Autodesk Fusion 360 part; units mm, degrees
(part 2 of 5)
sketch "Sketch7" plane through (0, 0, -0.05) normal (0, 0, -1) x (1, 0, 0)
  arc A0 (124.5324, 39.9718) -> (129.3118, 35.1924) centre (129.53, 40.19) ccw
  line L0 (129.3118, 35.1924) -> (129.53, 35.19)
  line L1 (129.53, 35.19) -> (210.09, 35.19)
  line L2 (210.09, 35.19) -> (210.3082, 35.1924)
  arc A1 (210.3082, 35.1924) -> (215.0876, 39.9718) centre (210.09, 40.19) ccw
  line L3 (215.0876, 39.9718) -> (215.09, 40.19)
  line L4 (215.09, 40.19) -> (215.09, 102.8)
  line L5 (215.09, 102.8) -> (215.0877, 103.0182)
  arc A2 (215.0877, 103.0182) -> (210.3082, 107.7977) centre (210.09, 102.8) ccw
  line L6 (210.3082, 107.7977) -> (210.09, 107.8)
  line L7 (210.09, 107.8) -> (129.53, 107.8)
  line L8 (129.53, 107.8) -> (129.3118, 107.7977)
  arc A3 (129.3118, 107.7977) -> (124.5323, 103.0182) centre (129.53, 102.8) ccw
  line L9 (124.5323, 103.0182) -> (124.53, 102.8)
  line L10 (124.53, 102.8) -> (124.53, 40.19)
  line L11 (124.53, 40.19) -> (124.5324, 39.9718)
  circle A4 centre (172, 103.08) radius 1.077
  circle A5 centre (184.5, 103.08) radius 1.077
  circle A6 centre (129.53, 102.8) radius 1.3
  circle A7 centre (210.09, 102.8) radius 1.3
  arc A8 (172.975, 97.003) -> (173.077, 97.105) centre (172.975, 97.105) ccw
  line L12 (172.975, 97.003) -> (171.025, 97.003)
  arc A9 (170.923, 97.105) -> (171.025, 97.003) centre (171.025, 97.105) ccw
  line L13 (170.923, 97.105) -> (170.923, 99.055)
  arc A10 (171.025, 99.157) -> (170.923, 99.055) centre (171.025, 99.055) ccw
  line L14 (171.025, 99.157) -> (172.975, 99.157)
  arc A11 (173.077, 99.055) -> (172.975, 99.157) centre (172.975, 99.055) ccw
  line L15 (173.077, 99.055) -> (173.077, 97.105)
  circle A12 centre (184.5, 98.08) radius 1.077
  line L16 (212.43, 78.91) -> (212.43, 77.21)
  line L17 (212.43, 77.21) -> (210.73, 77.21)
  line L18 (210.73, 77.21) -> (210.73, 78.91)
  line L19 (210.73, 78.91) -> (212.43, 78.91)
  circle A13 centre (211.58, 75.52) radius 0.85
  circle A14 centre (211.58, 72.98) radius 0.85
  circle A15 centre (211.58, 70.44) radius 0.85
  circle A16 centre (211.58, 67.9) radius 0.85
  circle A17 centre (211.58, 65.36) radius 0.85
  circle A18 centre (211.58, 62.82) radius 0.85
  circle A19 centre (211.58, 60.28) radius 0.85
  arc A20 (164.6391, 57.504) -> (164.7411, 57.606) centre (164.6391, 57.606) ccw
  line L20 (164.6391, 57.504) -> (162.6391, 57.504)
  arc A21 (162.5371, 57.606) -> (162.6391, 57.504) centre (162.6391, 57.606) ccw
  line L21 (162.5371, 57.606) -> (162.5371, 59.114)
  arc A22 (162.6391, 59.216) -> (162.5371, 59.114) centre (162.6391, 59.114) ccw
  line L22 (162.6391, 59.216) -> (164.6391, 59.216)
  arc A23 (164.7411, 59.114) -> (164.6391, 59.216) centre (164.6391, 59.114) ccw
  line L23 (164.7411, 59.114) -> (164.7411, 57.606)
  arc A24 (182.0197, 57.504) -> (182.1217, 57.606) centre (182.0197, 57.606) ccw
  line L24 (182.0197, 57.504) -> (180.0197, 57.504)
  arc A25 (179.9177, 57.606) -> (180.0197, 57.504) centre (180.0197, 57.606) ccw
  line L25 (179.9177, 57.606) -> (179.9177, 59.114)
  arc A26 (180.0197, 59.216) -> (179.9177, 59.114) centre (180.0197, 59.114) ccw
  line L26 (180.0197, 59.216) -> (182.0197, 59.216)
  arc A27 (182.1217, 59.114) -> (182.0197, 59.216) centre (182.0197, 59.114) ccw
  line L27 (182.1217, 59.114) -> (182.1217, 57.606)
  circle A28 centre (211.58, 57.74) radius 0.85
  arc A29 (164.6322, 54.964) -> (164.7342, 55.066) centre (164.6322, 55.066) ccw
  line L28 (164.6322, 54.964) -> (162.6322, 54.964)
  arc A30 (162.5302, 55.066) -> (162.6322, 54.964) centre (162.6322, 55.066) ccw
  line L29 (162.5302, 55.066) -> (162.5302, 56.574)
  arc A31 (162.6322, 56.676) -> (162.5302, 56.574) centre (162.6322, 56.574) ccw
  line L30 (162.6322, 56.676) -> (164.6322, 56.676)
  arc A32 (164.7342, 56.574) -> (164.6322, 56.676) centre (164.6322, 56.574) ccw
  line L31 (164.7342, 56.574) -> (164.7342, 55.066)
  arc A33 (182.0197, 54.964) -> (182.1217, 55.066) centre (182.0197, 55.066) ccw
  line L32 (182.0197, 54.964) -> (180.0197, 54.964)
  arc A34 (179.9177, 55.066) -> (180.0197, 54.964) centre (180.0197, 55.066) ccw
  line L33 (179.9177, 55.066) -> (179.9177, 56.574)
  arc A35 (180.0197, 56.676) -> (179.9177, 56.574) centre (180.0197, 56.574) ccw
  line L34 (180.0197, 56.676) -> (182.0197, 56.676)
  arc A36 (182.1217, 56.574) -> (182.0197, 56.676) centre (182.0197, 56.574) ccw
  line L35 (182.1217, 56.574) -> (182.1217, 55.066)
  circle A37 centre (211.58, 55.2) radius 0.85
  arc A38 (199.24, 52.73) -> (199.49, 52.98) centre (199.24, 52.98) ccw
  line L36 (199.24, 52.73) -> (198.59, 52.73)
  arc A39 (198.34, 52.98) -> (198.59, 52.73) centre (198.59, 52.98) ccw
  line L37 (198.34, 52.98) -> (198.34, 54.28)
  arc A40 (198.59, 54.53) -> (198.34, 54.28) centre (198.59, 54.28) ccw
  line L38 (198.59, 54.53) -> (199.24, 54.53)
  arc A41 (199.49, 54.28) -> (199.24, 54.53) centre (199.24, 54.28) ccw
  line L39 (199.49, 54.28) -> (199.49, 52.98)
  arc A42 (202.19, 52.73) -> (202.44, 52.98) centre (202.19, 52.98) ccw
  line L40 (202.19, 52.73) -> (201.54, 52.73)
  arc A43 (201.29, 52.98) -> (201.54, 52.73) centre (201.54, 52.98) ccw
  line L41 (201.29, 52.98) -> (201.29, 54.28)
  arc A44 (201.54, 54.53) -> (201.29, 54.28) centre (201.54, 54.28) ccw
  line L42 (201.54, 54.53) -> (202.19, 54.53)
  arc A45 (202.44, 54.28) -> (202.19, 54.53) centre (202.19, 54.28) ccw
  line L43 (202.44, 54.28) -> (202.44, 52.98)
  arc A46 (164.6322, 52.424) -> (164.7342, 52.526) centre (164.6322, 52.526) ccw
  line L44 (164.6322, 52.424) -> (162.6322, 52.424)
  arc A47 (162.5302, 52.526) -> (162.6322, 52.424) centre (162.6322, 52.526) ccw
  line L45 (162.5302, 52.526) -> (162.5302, 54.034)
  arc A48 (162.6322, 54.136) -> (162.5302, 54.034) centre (162.6322, 54.034) ccw
  line L46 (162.6322, 54.136) -> (164.6322, 54.136)
  arc A49 (164.7342, 54.034) -> (164.6322, 54.136) centre (164.6322, 54.034) ccw
  line L47 (164.7342, 54.034) -> (164.7342, 52.526)
  arc A50 (182.0197, 52.424) -> (182.1217, 52.526) centre (182.0197, 52.526) ccw
  line L48 (182.0197, 52.424) -> (180.0197, 52.424)
  arc A51 (179.9177, 52.526) -> (180.0197, 52.424) centre (180.0197, 52.526) ccw
  line L49 (179.9177, 52.526) -> (179.9177, 54.034)
  arc A52 (180.0197, 54.136) -> (179.9177, 54.034) centre (180.0197, 54.034) ccw
  line L50 (180.0197, 54.136) -> (182.0197, 54.136)
  arc A53 (182.1217, 54.034) -> (182.0197, 54.136) centre (182.0197, 54.034) ccw
  line L51 (182.1217, 54.034) -> (182.1217, 52.526)
  circle A54 centre (211.58, 52.66) radius 0.85
  arc A55 (164.6322, 49.884) -> (164.7342, 49.986) centre (164.6322, 49.986) ccw
  line L52 (164.6322, 49.884) -> (162.6322, 49.884)
  arc A56 (162.5302, 49.986) -> (162.6322, 49.884) centre (162.6322, 49.986) ccw
  line L53 (162.5302, 49.986) -> (162.5302, 51.494)
  arc A57 (162.6322, 51.596) -> (162.5302, 51.494) centre (162.6322, 51.494) ccw
  line L54 (162.6322, 51.596) -> (164.6322, 51.596)
  arc A58 (164.7342, 51.494) -> (164.6322, 51.596) centre (164.6322, 51.494) ccw
  line L55 (164.7342, 51.494) -> (164.7342, 49.986)
  arc A59 (182.0197, 49.884) -> (182.1217, 49.986) centre (182.0197, 49.986) ccw
  line L56 (182.0197, 49.884) -> (180.0197, 49.884)
  arc A60 (179.9177, 49.986) -> (180.0197, 49.884) centre (180.0197, 49.986) ccw
  line L57 (179.9177, 49.986) -> (179.9177, 51.494)
  arc A61 (180.0197, 51.596) -> (179.9177, 51.494) centre (180.0197, 51.494) ccw
  line L58 (180.0197, 51.596) -> (182.0197, 51.596)
  arc A62 (182.1217, 51.494) -> (182.0197, 51.596) centre (182.0197, 51.494) ccw
  line L59 (182.1217, 51.494) -> (182.1217, 49.986)
  line L60 (140.26, 51.04) -> (140.26, 49.44)
  line L61 (140.26, 49.44) -> (139.56, 49.44)
  line L62 (139.56, 49.44) -> (139.56, 51.04)
  line L63 (139.56, 51.04) -> (140.26, 51.04)
  line L64 (141.36, 51.04) -> (141.36, 49.44)
  line L65 (141.36, 49.44) -> (140.66, 49.44)
  line L66 (140.66, 49.44) -> (140.66, 51.04)
  line L67 (140.66, 51.04) -> (141.36, 51.04)
  line L68 (142.46, 51.04) -> (142.46, 49.44)
  line L69 (142.46, 49.44) -> (141.76, 49.44)
  line L70 (141.76, 49.44) -> (141.76, 51.04)
  line L71 (141.76, 51.04) -> (142.46, 51.04)
  line L72 (143.56, 51.04) -> (143.56, 49.44)
  line L73 (143.56, 49.44) -> (142.86, 49.44)
  line L74 (142.86, 49.44) -> (142.86, 51.04)
  line L75 (142.86, 51.04) -> (143.56, 51.04)
  line L76 (144.66, 51.04) -> (144.66, 49.44)
  line L77 (144.66, 49.44) -> (143.96, 49.44)
  line L78 (143.96, 49.44) -> (143.96, 51.04)
  line L79 (143.96, 51.04) -> (144.66, 51.04)
  line L80 (145.76, 51.04) -> (145.76, 49.44)
  line L81 (145.76, 49.44) -> (145.06, 49.44)
  line L82 (145.06, 49.44) -> (145.06, 51.04)
  line L83 (145.06, 51.04) -> (145.76, 51.04)
  line L84 (146.86, 51.04) -> (146.86, 49.44)
  line L85 (146.86, 49.44) -> (146.16, 49.44)
  line L86 (146.16, 49.44) -> (146.16, 51.04)
  line L87 (146.16, 51.04) -> (146.86, 51.04)
  line L88 (147.96, 51.04) -> (147.96, 49.44)
  line L89 (147.96, 49.44) -> (147.26, 49.44)
  line L90 (147.26, 49.44) -> (147.26, 51.04)
  line L91 (147.26, 51.04) -> (147.96, 51.04)
  line L92 (149.06, 51.04) -> (149.06, 49.44)
  line L93 (149.06, 49.44) -> (148.36, 49.44)
  line L94 (148.36, 49.44) -> (148.36, 51.04)
  line L95 (148.36, 51.04) -> (149.06, 51.04)
  circle A63 centre (211.58, 50.12) radius 0.85
  line L96 (139.26, 49.99) -> (139.26, 48.49)
  line L97 (139.26, 48.49) -> (138.06, 48.49)
  line L98 (138.06, 48.49) -> (138.06, 49.99)
  line L99 (138.06, 49.99) -> (139.26, 49.99)
  line L100 (154.11, 49.99) -> (154.11, 48.49)
  line L101 (154.11, 48.49) -> (152.51, 48.49)
  line L102 (152.51, 48.49) -> (152.51, 49.99)
  line L103 (152.51, 49.99) -> (154.11, 49.99)
  arc A64 (164.6322, 47.344) -> (164.7342, 47.446) centre (164.6322, 47.446) ccw
  line L104 (164.6322, 47.344) -> (162.6322, 47.344)
  arc A65 (162.5302, 47.446) -> (162.6322, 47.344) centre (162.6322, 47.446) ccw
  line L105 (162.5302, 47.446) -> (162.5302, 48.954)
  arc A66 (162.6322, 49.056) -> (162.5302, 48.954) centre (162.6322, 48.954) ccw
  line L106 (162.6322, 49.056) -> (164.6322, 49.056)
  arc A67 (164.7342, 48.954) -> (164.6322, 49.056) centre (164.6322, 48.954) ccw
  line L107 (164.7342, 48.954) -> (164.7342, 47.446)
  arc A68 (182.0197, 47.344) -> (182.1217, 47.446) centre (182.0197, 47.446) ccw
  line L108 (182.0197, 47.344) -> (180.0197, 47.344)
  arc A69 (179.9177, 47.446) -> (180.0197, 47.344) centre (180.0197, 47.446) ccw
  line L109 (179.9177, 47.446) -> (179.9177, 48.954)
  arc A70 (180.0197, 49.056) -> (179.9177, 48.954) centre (180.0197, 48.954) ccw
  line L110 (180.0197, 49.056) -> (182.0197, 49.056)
  arc A71 (182.1217, 48.954) -> (182.0197, 49.056) centre (182.0197, 48.954) ccw
  line L111 (182.1217, 48.954) -> (182.1217, 47.446)
  circle A72 centre (211.58, 47.58) radius 0.85
  circle A73 centre (196.89, 46.1501) radius 0.6604
  circle A74 centre (199.43, 46.1501) radius 0.6604
  circle A75 centre (201.97, 46.1501) radius 0.6604
  arc A76 (164.6322, 44.804) -> (164.7342, 44.906) centre (164.6322, 44.906) ccw
  line L112 (164.6322, 44.804) -> (162.6322, 44.804)
  arc A77 (162.5302, 44.906) -> (162.6322, 44.804) centre (162.6322, 44.906) ccw
  line L113 (162.5302, 44.906) -> (162.5302, 46.414)
  arc A78 (162.6322, 46.516) -> (162.5302, 46.414) centre (162.6322, 46.414) ccw
  line L114 (162.6322, 46.516) -> (164.6322, 46.516)
  arc A79 (164.7342, 46.414) -> (164.6322, 46.516) centre (164.6322, 46.414) ccw
  line L115 (164.7342, 46.414) -> (164.7342, 44.906)
  arc A80 (182.0197, 44.804) -> (182.1217, 44.906) centre (182.0197, 44.906) ccw
  line L116 (182.0197, 44.804) -> (180.0197, 44.804)
  arc A81 (179.9177, 44.906) -> (180.0197, 44.804) centre (180.0197, 44.906) ccw
  line L117 (179.9177, 44.906) -> (179.9177, 46.414)
  arc A82 (180.0197, 46.516) -> (179.9177, 46.414) centre (180.0197, 46.414) ccw
  line L118 (180.0197, 46.516) -> (182.0197, 46.516)
  arc A83 (182.1217, 46.414) -> (182.0197, 46.516) centre (182.0197, 46.414) ccw
  line L119 (182.1217, 46.414) -> (182.1217, 44.906)
  circle A84 centre (211.58, 45.04) radius 0.85
  arc A85 (164.6322, 42.264) -> (164.7342, 42.366) centre (164.6322, 42.366) ccw
  line L120 (164.6322, 42.264) -> (162.6322, 42.264)
  arc A86 (162.5302, 42.366) -> (162.6322, 42.264) centre (162.6322, 42.366) ccw
  line L121 (162.5302, 42.366) -> (162.5302, 43.874)
  arc A87 (162.6322, 43.976) -> (162.5302, 43.874) centre (162.6322, 43.874) ccw
  line L122 (162.6322, 43.976) -> (164.6322, 43.976)
  arc A88 (164.7342, 43.874) -> (164.6322, 43.976) centre (164.6322, 43.874) ccw
  line L123 (164.7342, 43.874) -> (164.7342, 42.366)
  arc A89 (182.0197, 42.264) -> (182.1217, 42.366) centre (182.0197, 42.366) ccw
  line L124 (182.0197, 42.264) -> (180.0197, 42.264)
  arc A90 (179.9177, 42.366) -> (180.0197, 42.264) centre (180.0197, 42.366) ccw
  line L125 (179.9177, 42.366) -> (179.9177, 43.874)
  arc A91 (180.0197, 43.976) -> (179.9177, 43.874) centre (180.0197, 43.874) ccw
  line L126 (180.0197, 43.976) -> (182.0197, 43.976)
  arc A92 (182.1217, 43.874) -> (182.0197, 43.976) centre (182.0197, 43.874) ccw
  line L127 (182.1217, 43.874) -> (182.1217, 42.366)
  circle A93 centre (129.53, 40.19) radius 1.3
  circle A94 centre (210.09, 40.19) radius 1.3
  arc A95 (164.6322, 39.724) -> (164.7342, 39.826) centre (164.6322, 39.826) ccw
  line L128 (164.6322, 39.724) -> (162.6322, 39.724)
  arc A96 (162.5302, 39.826) -> (162.6322, 39.724) centre (162.6322, 39.826) ccw
  line L129 (162.5302, 39.826) -> (162.5302, 41.334)
  arc A97 (162.6322, 41.436) -> (162.5302, 41.334) centre (162.6322, 41.334) ccw
  line L130 (162.6322, 41.436) -> (164.6322, 41.436)
  arc A98 (164.7342, 41.334) -> (164.6322, 41.436) centre (164.6322, 41.334) ccw
  line L131 (164.7342, 41.334) -> (164.7342, 39.826)
  arc A99 (182.0197, 39.724) -> (182.1217, 39.826) centre (182.0197, 39.826) ccw
  line L132 (182.0197, 39.724) -> (180.0197, 39.724)
  arc A100 (179.9177, 39.826) -> (180.0197, 39.724) centre (180.0197, 39.826) ccw
  line L133 (179.9177, 39.826) -> (179.9177, 41.334)
  arc A101 (180.0197, 41.436) -> (179.9177, 41.334) centre (180.0197, 41.334) ccw
  line L134 (180.0197, 41.436) -> (182.0197, 41.436)
  arc A102 (182.1217, 41.334) -> (182.0197, 41.436) centre (182.0197, 41.334) ccw
  line L135 (182.1217, 41.334) -> (182.1217, 39.826)
  line L136 (139.26, 40.74) -> (139.26, 38.54)
  line L137 (139.26, 38.54) -> (138.06, 38.54)
  line L138 (138.06, 38.54) -> (138.06, 40.74)
  line L139 (138.06, 40.74) -> (139.26, 40.74)
  line L140 (154.86, 40.74) -> (154.86, 38.54)
  line L141 (154.86, 38.54) -> (153.66, 38.54)
  line L142 (153.66, 38.54) -> (153.66, 40.74)
  line L143 (153.66, 40.74) -> (154.86, 40.74)
  arc A103 (164.6322, 37.184) -> (164.7342, 37.286) centre (164.6322, 37.286) ccw
  line L144 (164.6322, 37.184) -> (162.6322, 37.184)
  arc A104 (162.5302, 37.286) -> (162.6322, 37.184) centre (162.6322, 37.286) ccw
  line L145 (162.5302, 37.286) -> (162.5302, 38.794)
  arc A105 (162.6322, 38.896) -> (162.5302, 38.794) centre (162.6322, 38.794) ccw
  line L146 (162.6322, 38.896) -> (164.6322, 38.896)
  arc A106 (164.7342, 38.794) -> (164.6322, 38.896) centre (164.6322, 38.794) ccw
  line L147 (164.7342, 38.794) -> (164.7342, 37.286)
  arc A107 (182.0197, 37.184) -> (182.1217, 37.286) centre (182.0197, 37.286) ccw
  line L148 (182.0197, 37.184) -> (180.0197, 37.184)
  arc A108 (179.9177, 37.286) -> (180.0197, 37.184) centre (180.0197, 37.286) ccw
  line L149 (179.9177, 37.286) -> (179.9177, 38.794)
  arc A109 (180.0197, 38.896) -> (179.9177, 38.794) centre (180.0197, 38.794) ccw
  line L150 (180.0197, 38.896) -> (182.0197, 38.896)
  arc A110 (182.1217, 38.794) -> (182.0197, 38.896) centre (182.0197, 38.794) ccw
  line L151 (182.1217, 38.794) -> (182.1217, 37.286)
  circle A111 centre (129.53, 102.8) radius 6.8089
  circle A112 centre (129.53, 40.19) radius 7.6352
  spline S0 degree 5 poles (207.5436, 38.5257) (207.5062, 38.7717) (207.4443, 39.2717) (207.3918, 40.0335) (207.4207, 41.0207) (207.6971, 42.0707) (208.2833, 42.8142) (209.2088, 43.1592) (210.4206, 43.0662) (211.7646, 42.5596) (213.0388, 41.708) (214.0308, 40.6116) (214.5637, 39.3872) (214.5339, 38.1559) (213.9669, 37.0286) (212.9954, 36.1) (211.807, 35.4469) (210.6011, 35.1248) (209.5472, 35.1641) (208.7311, 35.5656) (208.1502, 36.299) (207.8391, 37.1051) (207.6691, 37.7955) (207.5811, 38.2796) (207.5436, 38.5257) knots 0 0 0 0 0 0 0.05 0.1 0.15 0.2 0.25 0.3 0.35 0.4 0.45 0.5 0.55 0.6 0.65 0.7 0.75 0.8 0.85 0.9 0.95 1 1 1 1 1 1
  point P0 (209, 43)
  point P1 (214.4745, 39.0133)
  point P2 (210.09, 35.19)
  constraint concentric A3 A111
  constraint concentric A0 A112
  constraint coincident P2 L1.end
extrude "Extrude6" add sketch "Sketch7" along normal blind 20.6 contours L2 A1 S0 | A94 picked at (207.9612, 39.4019)
sketch "Sketch8" plane through (0, 0, -0.05) normal (0, 0, -1) x (1, 0, 0)
  arc A0 (124.5324, 39.9718) -> (129.3118, 35.1924) centre (129.53, 40.19) ccw
  line L0 (129.3118, 35.1924) -> (129.53, 35.19)
  line L1 (129.53, 35.19) -> (210.09, 35.19)
  line L2 (210.09, 35.19) -> (210.3082, 35.1924)
  arc A1 (210.3082, 35.1924) -> (215.0876, 39.9718) centre (210.09, 40.19) ccw
  line L3 (215.0876, 39.9718) -> (215.09, 40.19)
  line L4 (215.09, 40.19) -> (215.09, 102.8)
  line L5 (215.09, 102.8) -> (215.0877, 103.0182)
  arc A2 (215.0877, 103.0182) -> (210.3082, 107.7977) centre (210.09, 102.8) ccw
  line L6 (210.3082, 107.7977) -> (210.09, 107.8)
  line L7 (210.09, 107.8) -> (129.53, 107.8)
  line L8 (129.53, 107.8) -> (129.3118, 107.7977)
  arc A3 (129.3118, 107.7977) -> (124.5323, 103.0182) centre (129.53, 102.8) ccw
  line L9 (124.5323, 103.0182) -> (124.53, 102.8)
  line L10 (124.53, 102.8) -> (124.53, 40.19)
  line L11 (124.53, 40.19) -> (124.5324, 39.9718)
  circle A4 centre (172, 103.08) radius 1.077
  circle A5 centre (184.5, 103.08) radius 1.077
  circle A6 centre (129.53, 102.8) radius 1.3
  circle A7 centre (210.09, 102.8) radius 1.3
  arc A8 (172.975, 97.003) -> (173.077, 97.105) centre (172.975, 97.105) ccw
  line L12 (172.975, 97.003) -> (171.025, 97.003)
  arc A9 (170.923, 97.105) -> (171.025, 97.003) centre (171.025, 97.105) ccw
  line L13 (170.923, 97.105) -> (170.923, 99.055)
  arc A10 (171.025, 99.157) -> (170.923, 99.055) centre (171.025, 99.055) ccw
  line L14 (171.025, 99.157) -> (172.975, 99.157)
  arc A11 (173.077, 99.055) -> (172.975, 99.157) centre (172.975, 99.055) ccw
  line L15 (173.077, 99.055) -> (173.077, 97.105)
  circle A12 centre (184.5, 98.08) radius 1.077
  line L16 (212.43, 78.91) -> (212.43, 77.21)
  line L17 (212.43, 77.21) -> (210.73, 77.21)
  line L18 (210.73, 77.21) -> (210.73, 78.91)
  line L19 (210.73, 78.91) -> (212.43, 78.91)
  circle A13 centre (211.58, 75.52) radius 0.85
  circle A14 centre (211.58, 72.98) radius 0.85
  circle A15 centre (211.58, 70.44) radius 0.85
  circle A16 centre (211.58, 67.9) radius 0.85
  circle A17 centre (211.58, 65.36) radius 0.85
  circle A18 centre (211.58, 62.82) radius 0.85
  circle A19 centre (211.58, 60.28) radius 0.85
  arc A20 (164.6391, 57.504) -> (164.7411, 57.606) centre (164.6391, 57.606) ccw
  line L20 (164.6391, 57.504) -> (162.6391, 57.504)
  arc A21 (162.5371, 57.606) -> (162.6391, 57.504) centre (162.6391, 57.606) ccw
  line L21 (162.5371, 57.606) -> (162.5371, 59.114)
  arc A22 (162.6391, 59.216) -> (162.5371, 59.114) centre (162.6391, 59.114) ccw
  line L22 (162.6391, 59.216) -> (164.6391, 59.216)
  arc A23 (164.7411, 59.114) -> (164.6391, 59.216) centre (164.6391, 59.114) ccw
  line L23 (164.7411, 59.114) -> (164.7411, 57.606)
  arc A24 (182.0197, 57.504) -> (182.1217, 57.606) centre (182.0197, 57.606) ccw
  line L24 (182.0197, 57.504) -> (180.0197, 57.504)
  arc A25 (179.9177, 57.606) -> (180.0197, 57.504) centre (180.0197, 57.606) ccw
  line L25 (179.9177, 57.606) -> (179.9177, 59.114)
  arc A26 (180.0197, 59.216) -> (179.9177, 59.114) centre (180.0197, 59.114) ccw
  line L26 (180.0197, 59.216) -> (182.0197, 59.216)
  arc A27 (182.1217, 59.114) -> (182.0197, 59.216) centre (182.0197, 59.114) ccw
  line L27 (182.1217, 59.114) -> (182.1217, 57.606)
  circle A28 centre (211.58, 57.74) radius 0.85
  arc A29 (164.6322, 54.964) -> (164.7342, 55.066) centre (164.6322, 55.066) ccw
  line L28 (164.6322, 54.964) -> (162.6322, 54.964)
  arc A30 (162.5302, 55.066) -> (162.6322, 54.964) centre (162.6322, 55.066) ccw
  line L29 (162.5302, 55.066) -> (162.5302, 56.574)
  arc A31 (162.6322, 56.676) -> (162.5302, 56.574) centre (162.6322, 56.574) ccw
  line L30 (162.6322, 56.676) -> (164.6322, 56.676)
  arc A32 (164.7342, 56.574) -> (164.6322, 56.676) centre (164.6322, 56.574) ccw
  line L31 (164.7342, 56.574) -> (164.7342, 55.066)
  arc A33 (182.0197, 54.964) -> (182.1217, 55.066) centre (182.0197, 55.066) ccw
  line L32 (182.0197, 54.964) -> (180.0197, 54.964)
  arc A34 (179.9177, 55.066) -> (180.0197, 54.964) centre (180.0197, 55.066) ccw
  line L33 (179.9177, 55.066) -> (179.9177, 56.574)
  arc A35 (180.0197, 56.676) -> (179.9177, 56.574) centre (180.0197, 56.574) ccw
  line L34 (180.0197, 56.676) -> (182.0197, 56.676)
  arc A36 (182.1217, 56.574) -> (182.0197, 56.676) centre (182.0197, 56.574) ccw
  line L35 (182.1217, 56.574) -> (182.1217, 55.066)
  circle A37 centre (211.58, 55.2) radius 0.85
  arc A38 (199.24, 52.73) -> (199.49, 52.98) centre (199.24, 52.98) ccw
  line L36 (199.24, 52.73) -> (198.59, 52.73)
  arc A39 (198.34, 52.98) -> (198.59, 52.73) centre (198.59, 52.98) ccw
  line L37 (198.34, 52.98) -> (198.34, 54.28)
  arc A40 (198.59, 54.53) -> (198.34, 54.28) centre (198.59, 54.28) ccw
  line L38 (198.59, 54.53) -> (199.24, 54.53)
  arc A41 (199.49, 54.28) -> (199.24, 54.53) centre (199.24, 54.28) ccw
  line L39 (199.49, 54.28) -> (199.49, 52.98)
  arc A42 (202.19, 52.73) -> (202.44, 52.98) centre (202.19, 52.98) ccw
  line L40 (202.19, 52.73) -> (201.54, 52.73)
  arc A43 (201.29, 52.98) -> (201.54, 52.73) centre (201.54, 52.98) ccw
  line L41 (201.29, 52.98) -> (201.29, 54.28)
  arc A44 (201.54, 54.53) -> (201.29, 54.28) centre (201.54, 54.28) ccw
  line L42 (201.54, 54.53) -> (202.19, 54.53)
  arc A45 (202.44, 54.28) -> (202.19, 54.53) centre (202.19, 54.28) ccw
  line L43 (202.44, 54.28) -> (202.44, 52.98)
  arc A46 (164.6322, 52.424) -> (164.7342, 52.526) centre (164.6322, 52.526) ccw
  line L44 (164.6322, 52.424) -> (162.6322, 52.424)
  arc A47 (162.5302, 52.526) -> (162.6322, 52.424) centre (162.6322, 52.526) ccw
  line L45 (162.5302, 52.526) -> (162.5302, 54.034)
  arc A48 (162.6322, 54.136) -> (162.5302, 54.034) centre (162.6322, 54.034) ccw
  line L46 (162.6322, 54.136) -> (164.6322, 54.136)
  arc A49 (164.7342, 54.034) -> (164.6322, 54.136) centre (164.6322, 54.034) ccw
  line L47 (164.7342, 54.034) -> (164.7342, 52.526)
  arc A50 (182.0197, 52.424) -> (182.1217, 52.526) centre (182.0197, 52.526) ccw
  line L48 (182.0197, 52.424) -> (180.0197, 52.424)
  arc A51 (179.9177, 52.526) -> (180.0197, 52.424) centre (180.0197, 52.526) ccw
  line L49 (179.9177, 52.526) -> (179.9177, 54.034)
  arc A52 (180.0197, 54.136) -> (179.9177, 54.034) centre (180.0197, 54.034) ccw
  line L50 (180.0197, 54.136) -> (182.0197, 54.136)
  arc A53 (182.1217, 54.034) -> (182.0197, 54.136) centre (182.0197, 54.034) ccw
  line L51 (182.1217, 54.034) -> (182.1217, 52.526)
  circle A54 centre (211.58, 52.66) radius 0.85
  arc A55 (164.6322, 49.884) -> (164.7342, 49.986) centre (164.6322, 49.986) ccw
  line L52 (164.6322, 49.884) -> (162.6322, 49.884)
  arc A56 (162.5302, 49.986) -> (162.6322, 49.884) centre (162.6322, 49.986) ccw
  line L53 (162.5302, 49.986) -> (162.5302, 51.494)
  arc A57 (162.6322, 51.596) -> (162.5302, 51.494) centre (162.6322, 51.494) ccw
  line L54 (162.6322, 51.596) -> (164.6322, 51.596)
  arc A58 (164.7342, 51.494) -> (164.6322, 51.596) centre (164.6322, 51.494) ccw
  line L55 (164.7342, 51.494) -> (164.7342, 49.986)
  arc A59 (182.0197, 49.884) -> (182.1217, 49.986) centre (182.0197, 49.986) ccw
  line L56 (182.0197, 49.884) -> (180.0197, 49.884)
  arc A60 (179.9177, 49.986) -> (180.0197, 49.884) centre (180.0197, 49.986) ccw
  line L57 (179.9177, 49.986) -> (179.9177, 51.494)
  arc A61 (180.0197, 51.596) -> (179.9177, 51.494) centre (180.0197, 51.494) ccw
  line L58 (180.0197, 51.596) -> (182.0197, 51.596)
  arc A62 (182.1217, 51.494) -> (182.0197, 51.596) centre (182.0197, 51.494) ccw
  line L59 (182.1217, 51.494) -> (182.1217, 49.986)
  line L60 (140.26, 51.04) -> (140.26, 49.44)
  line L61 (140.26, 49.44) -> (139.56, 49.44)
  line L62 (139.56, 49.44) -> (139.56, 51.04)
  line L63 (139.56, 51.04) -> (140.26, 51.04)
  line L64 (141.36, 51.04) -> (141.36, 49.44)
  line L65 (141.36, 49.44) -> (140.66, 49.44)
  line L66 (140.66, 49.44) -> (140.66, 51.04)
  line L67 (140.66, 51.04) -> (141.36, 51.04)
  line L68 (142.46, 51.04) -> (142.46, 49.44)
  line L69 (142.46, 49.44) -> (141.76, 49.44)
  line L70 (141.76, 49.44) -> (141.76, 51.04)
  line L71 (141.76, 51.04) -> (142.46, 51.04)
  line L72 (143.56, 51.04) -> (143.56, 49.44)
  line L73 (143.56, 49.44) -> (142.86, 49.44)
  line L74 (142.86, 49.44) -> (142.86, 51.04)
  line L75 (142.86, 51.04) -> (143.56, 51.04)
  line L76 (144.66, 51.04) -> (144.66, 49.44)
  line L77 (144.66, 49.44) -> (143.96, 49.44)
  line L78 (143.96, 49.44) -> (143.96, 51.04)
  line L79 (143.96, 51.04) -> (144.66, 51.04)
  line L80 (145.76, 51.04) -> (145.76, 49.44)
  line L81 (145.76, 49.44) -> (145.06, 49.44)
  line L82 (145.06, 49.44) -> (145.06, 51.04)
  line L83 (145.06, 51.04) -> (145.76, 51.04)
  line L84 (146.86, 51.04) -> (146.86, 49.44)
  line L85 (146.86, 49.44) -> (146.16, 49.44)
  line L86 (146.16, 49.44) -> (146.16, 51.04)
  line L87 (146.16, 51.04) -> (146.86, 51.04)
  line L88 (147.96, 51.04) -> (147.96, 49.44)
  line L89 (147.96, 49.44) -> (147.26, 49.44)
  line L90 (147.26, 49.44) -> (147.26, 51.04)
  line L91 (147.26, 51.04) -> (147.96, 51.04)
  line L92 (149.06, 51.04) -> (149.06, 49.44)
  line L93 (149.06, 49.44) -> (148.36, 49.44)
  line L94 (148.36, 49.44) -> (148.36, 51.04)
  line L95 (148.36, 51.04) -> (149.06, 51.04)
  circle A63 centre (211.58, 50.12) radius 0.85
  line L96 (139.26, 49.99) -> (139.26, 48.49)
  line L97 (139.26, 48.49) -> (138.06, 48.49)
  line L98 (138.06, 48.49) -> (138.06, 49.99)
  line L99 (138.06, 49.99) -> (139.26, 49.99)
  line L100 (154.11, 49.99) -> (154.11, 48.49)
  line L101 (154.11, 48.49) -> (152.51, 48.49)
  line L102 (152.51, 48.49) -> (152.51, 49.99)
  line L103 (152.51, 49.99) -> (154.11, 49.99)
  arc A64 (164.6322, 47.344) -> (164.7342, 47.446) centre (164.6322, 47.446) ccw
  line L104 (164.6322, 47.344) -> (162.6322, 47.344)
  arc A65 (162.5302, 47.446) -> (162.6322, 47.344) centre (162.6322, 47.446) ccw
  line L105 (162.5302, 47.446) -> (162.5302, 48.954)
  arc A66 (162.6322, 49.056) -> (162.5302, 48.954) centre (162.6322, 48.954) ccw
  line L106 (162.6322, 49.056) -> (164.6322, 49.056)
  arc A67 (164.7342, 48.954) -> (164.6322, 49.056) centre (164.6322, 48.954) ccw
  line L107 (164.7342, 48.954) -> (164.7342, 47.446)
  arc A68 (182.0197, 47.344) -> (182.1217, 47.446) centre (182.0197, 47.446) ccw
  line L108 (182.0197, 47.344) -> (180.0197, 47.344)
  arc A69 (179.9177, 47.446) -> (180.0197, 47.344) centre (180.0197, 47.446) ccw
  line L109 (179.9177, 47.446) -> (179.9177, 48.954)
  arc A70 (180.0197, 49.056) -> (179.9177, 48.954) centre (180.0197, 48.954) ccw
  line L110 (180.0197, 49.056) -> (182.0197, 49.056)
  arc A71 (182.1217, 48.954) -> (182.0197, 49.056) centre (182.0197, 48.954) ccw
  line L111 (182.1217, 48.954) -> (182.1217, 47.446)
  circle A72 centre (211.58, 47.58) radius 0.85
  circle A73 centre (196.89, 46.1501) radius 0.6604
  circle A74 centre (199.43, 46.1501) radius 0.6604
  circle A75 centre (201.97, 46.1501) radius 0.6604
  arc A76 (164.6322, 44.804) -> (164.7342, 44.906) centre (164.6322, 44.906) ccw
  line L112 (164.6322, 44.804) -> (162.6322, 44.804)
  arc A77 (162.5302, 44.906) -> (162.6322, 44.804) centre (162.6322, 44.906) ccw
  line L113 (162.5302, 44.906) -> (162.5302, 46.414)
  arc A78 (162.6322, 46.516) -> (162.5302, 46.414) centre (162.6322, 46.414) ccw
  line L114 (162.6322, 46.516) -> (164.6322, 46.516)
  arc A79 (164.7342, 46.414) -> (164.6322, 46.516) centre (164.6322, 46.414) ccw
  line L115 (164.7342, 46.414) -> (164.7342, 44.906)
  arc A80 (182.0197, 44.804) -> (182.1217, 44.906) centre (182.0197, 44.906) ccw
  line L116 (182.0197, 44.804) -> (180.0197, 44.804)
  arc A81 (179.9177, 44.906) -> (180.0197, 44.804) centre (180.0197, 44.906) ccw
  line L117 (179.9177, 44.906) -> (179.9177, 46.414)
  arc A82 (180.0197, 46.516) -> (179.9177, 46.414) centre (180.0197, 46.414) ccw
  line L118 (180.0197, 46.516) -> (182.0197, 46.516)
  arc A83 (182.1217, 46.414) -> (182.0197, 46.516) centre (182.0197, 46.414) ccw
  line L119 (182.1217, 46.414) -> (182.1217, 44.906)
  circle A84 centre (211.58, 45.04) radius 0.85
  arc A85 (164.6322, 42.264) -> (164.7342, 42.366) centre (164.6322, 42.366) ccw
  line L120 (164.6322, 42.264) -> (162.6322, 42.264)
  arc A86 (162.5302, 42.366) -> (162.6322, 42.264) centre (162.6322, 42.366) ccw
  line L121 (162.5302, 42.366) -> (162.5302, 43.874)
  arc A87 (162.6322, 43.976) -> (162.5302, 43.874) centre (162.6322, 43.874) ccw
  line L122 (162.6322, 43.976) -> (164.6322, 43.976)
  arc A88 (164.7342, 43.874) -> (164.6322, 43.976) centre (164.6322, 43.874) ccw
  line L123 (164.7342, 43.874) -> (164.7342, 42.366)
  arc A89 (182.0197, 42.264) -> (182.1217, 42.366) centre (182.0197, 42.366) ccw
  line L124 (182.0197, 42.264) -> (180.0197, 42.264)
  arc A90 (179.9177, 42.366) -> (180.0197, 42.264) centre (180.0197, 42.366) ccw
  line L125 (179.9177, 42.366) -> (179.9177, 43.874)
  arc A91 (180.0197, 43.976) -> (179.9177, 43.874) centre (180.0197, 43.874) ccw
  line L126 (180.0197, 43.976) -> (182.0197, 43.976)
  arc A92 (182.1217, 43.874) -> (182.0197, 43.976) centre (182.0197, 43.874) ccw
  line L127 (182.1217, 43.874) -> (182.1217, 42.366)
  circle A93 centre (129.53, 40.19) radius 1.3
  circle A94 centre (210.09, 40.19) radius 1.3
  arc A95 (164.6322, 39.724) -> (164.7342, 39.826) centre (164.6322, 39.826) ccw
  line L128 (164.6322, 39.724) -> (162.6322, 39.724)
  arc A96 (162.5302, 39.826) -> (162.6322, 39.724) centre (162.6322, 39.826) ccw
  line L129 (162.5302, 39.826) -> (162.5302, 41.334)
  arc A97 (162.6322, 41.436) -> (162.5302, 41.334) centre (162.6322, 41.334) ccw
  line L130 (162.6322, 41.436) -> (164.6322, 41.436)
  arc A98 (164.7342, 41.334) -> (164.6322, 41.436) centre (164.6322, 41.334) ccw
  line L131 (164.7342, 41.334) -> (164.7342, 39.826)
  arc A99 (182.0197, 39.724) -> (182.1217, 39.826) centre (182.0197, 39.826) ccw
  line L132 (182.0197, 39.724) -> (180.0197, 39.724)
  arc A100 (179.9177, 39.826) -> (180.0197, 39.724) centre (180.0197, 39.826) ccw
  line L133 (179.9177, 39.826) -> (179.9177, 41.334)
  arc A101 (180.0197, 41.436) -> (179.9177, 41.334) centre (180.0197, 41.334) ccw
  line L134 (180.0197, 41.436) -> (182.0197, 41.436)
  arc A102 (182.1217, 41.334) -> (182.0197, 41.436) centre (182.0197, 41.334) ccw
  line L135 (182.1217, 41.334) -> (182.1217, 39.826)
  line L136 (139.26, 40.74) -> (139.26, 38.54)
  line L137 (139.26, 38.54) -> (138.06, 38.54)
  line L138 (138.06, 38.54) -> (138.06, 40.74)
  line L139 (138.06, 40.74) -> (139.26, 40.74)
  line L140 (154.86, 40.74) -> (154.86, 38.54)
  line L141 (154.86, 38.54) -> (153.66, 38.54)
  line L142 (153.66, 38.54) -> (153.66, 40.74)
  line L143 (153.66, 40.74) -> (154.86, 40.74)
  arc A103 (164.6322, 37.184) -> (164.7342, 37.286) centre (164.6322, 37.286) ccw
  line L144 (164.6322, 37.184) -> (162.6322, 37.184)
  arc A104 (162.5302, 37.286) -> (162.6322, 37.184) centre (162.6322, 37.286) ccw
  line L145 (162.5302, 37.286) -> (162.5302, 38.794)
  arc A105 (162.6322, 38.896) -> (162.5302, 38.794) centre (162.6322, 38.794) ccw
  line L146 (162.6322, 38.896) -> (164.6322, 38.896)
  arc A106 (164.7342, 38.794) -> (164.6322, 38.896) centre (164.6322, 38.794) ccw
  line L147 (164.7342, 38.794) -> (164.7342, 37.286)
  arc A107 (182.0197, 37.184) -> (182.1217, 37.286) centre (182.0197, 37.286) ccw
  line L148 (182.0197, 37.184) -> (180.0197, 37.184)
  arc A108 (179.9177, 37.286) -> (180.0197, 37.184) centre (180.0197, 37.286) ccw
  line L149 (179.9177, 37.286) -> (179.9177, 38.794)
  arc A109 (180.0197, 38.896) -> (179.9177, 38.794) centre (180.0197, 38.794) ccw
  line L150 (180.0197, 38.896) -> (182.0197, 38.896)
  arc A110 (182.1217, 38.794) -> (182.0197, 38.896) centre (182.0197, 38.794) ccw
  line L151 (182.1217, 38.794) -> (182.1217, 37.286)
  circle A111 centre (129.53, 102.8) radius 8.918
  constraint concentric A6 A111
extrude "Extrude7" add sketch "Sketch8" along normal blind 20.6 contours L7 L8 A3 L9 L10 A111 | A6 picked at (132.3092, 106.4281)
sketch "Sketch9" plane through (0, -28.19, 0) normal (0, 1, 0) x (-1, 0, 0)
  line L0 (-193.7671, -13.9329) -> (-205.2267, -13.9329)
  line L1 (-205.2267, -13.9329) -> (-205.2267, -0.4907)
  line L2 (-205.2267, -0.4907) -> (-193.7671, -0.4907)
  line L3 (-193.7671, -0.4907) -> (-193.7671, -13.9329)
  line L4 (-178.5005, -5.7083) -> (-179.0241, -4.7921)
  line L5 (-179.0241, -4.7921) -> (-179.1861, -3.8201)
  line L6 (-179.1861, -3.8201) -> (-179.0982, -2.4144)
  line L7 (-179.0982, -2.4144) -> (-178.5967, -1.0576)
  line L8 (-178.5967, -1.0576) -> (-177.2431, 0.1341)
  line L9 (-177.2431, 0.1341) -> (-175.9505, 0.474)
  line L10 (-175.9505, 0.474) -> (-168.8924, 0.474)
  line L11 (-168.8924, 0.474) -> (-167.3963, 0.0024)
  line L12 (-167.3963, 0.0024) -> (-166.4856, -0.9319)
  line L13 (-166.4856, -0.9319) -> (-165.8806, -1.8394)
  line L14 (-165.8806, -1.8394) -> (-165.7303, -2.8217)
  line L15 (-165.7303, -2.8217) -> (-165.7303, -3.8535)
  line L16 (-165.7303, -3.8535) -> (-165.8554, -4.7959)
  line L17 (-165.8554, -4.7959) -> (-166.3626, -5.6931)
  line L18 (-166.3626, -5.6931) -> (-167.1889, -6.6442)
  line L19 (-167.1889, -6.6442) -> (-168.8534, -7.2226)
  line L20 (-168.8534, -7.2226) -> (-176.0475, -7.2226)
  line L21 (-176.0475, -7.2226) -> (-177.5801, -6.7537)
  line L22 (-177.5801, -6.7537) -> (-178.5005, -5.7083)
  line L23 (-136.6822, 1.56) -> (-136.6822, -4.3178)
  line L24 (-136.6822, -4.3178) -> (-156.1178, -4.3178)
  line L25 (-156.1178, -4.3178) -> (-156.1178, 1.56)
  line L26 (-156.1178, 1.56) -> (-210.1282, 1.56)
  line L27 (-210.1282, 1.56) -> (-210.1282, -20.44)
  line L28 (-210.1282, -20.44) -> (-129.4918, -20.44)
  line L29 (-129.4918, -20.44) -> (-129.4918, 1.56)
  line L30 (-129.4918, 1.56) -> (-136.6822, 1.56)
  line L31 (-205.2267, -0.4907) -> (-193.7671, -0.4907)
  line L32 (-193.7671, -0.4907) -> (-193.7671, -13.9329)
  line L33 (-193.7671, -13.9329) -> (-205.2267, -13.9329)
  line L34 (-205.2267, -13.9329) -> (-205.2267, -0.4907)
  line L35 (-193.2554, -14.4446) -> (-205.7384, -14.4446)
  line L36 (-205.7384, -14.4446) -> (-205.7384, 0.0211)
  line L37 (-205.7384, 0.0211) -> (-193.2554, 0.0211)
  line L38 (-193.2554, 0.0211) -> (-193.2554, -14.4446)
  dimension "d19" = -0.5117
  constraint horizontal L31
  constraint vertical L32
  constraint horizontal L33
  constraint vertical L34
  constraint coincident L0.start L3.end
  constraint coincident L1.end L2.start
extrude "Extrude8" cut sketch "Sketch9" against normal blind 8 contours L35 L36 L37 L38
extrude "Extrude9" cut sketch "Sketch5" against normal blind 4.5 contours A32
sketch "Sketch10" plane through (0, 0, 1.56) normal (0, 0, 1) x (-1, 0, 0)
  arc A0 (-129.3118, 35.1924) -> (-124.5324, 39.9718) centre (-129.53, 40.19) ccw
  line L0 (-124.5324, 39.9718) -> (-124.53, 40.19)
  line L1 (-124.53, 40.19) -> (-124.53, 102.8)
  line L2 (-124.53, 102.8) -> (-124.5323, 103.0182)
  arc A1 (-124.5323, 103.0182) -> (-129.3118, 107.7977) centre (-129.53, 102.8) ccw
  line L3 (-129.3118, 107.7977) -> (-129.53, 107.8)
  line L4 (-129.53, 107.8) -> (-210.09, 107.8)
  line L5 (-210.09, 107.8) -> (-210.3082, 107.7977)
  arc A2 (-210.3082, 107.7977) -> (-215.0877, 103.0182) centre (-210.09, 102.8) ccw
  line L6 (-215.0877, 103.0182) -> (-215.09, 102.8)
  line L7 (-215.09, 102.8) -> (-215.09, 40.19)
  line L8 (-215.09, 40.19) -> (-215.0876, 39.9718)
  arc A3 (-215.0876, 39.9718) -> (-210.3082, 35.1924) centre (-210.09, 40.19) ccw
  line L9 (-210.3082, 35.1924) -> (-210.09, 35.19)
  line L10 (-210.09, 35.19) -> (-129.53, 35.19)
  line L11 (-129.53, 35.19) -> (-129.3118, 35.1924)
  circle A4 centre (-129.53, 102.8) radius 2.2
  circle A5 centre (-210.09, 102.8) radius 2.2
  line L12 (-153, 103.32) -> (-153, 104.72)
  line L13 (-153, 104.72) -> (-151, 104.72)
  line L14 (-151, 104.72) -> (-151, 103.32)
  line L15 (-151, 103.32) -> (-153, 103.32)
  line L16 (-164.46, 103.32) -> (-164.46, 104.72)
  line L17 (-164.46, 104.72) -> (-162.46, 104.72)
  line L18 (-162.46, 104.72) -> (-162.46, 103.32)
  line L19 (-162.46, 103.32) -> (-164.46, 103.32)
  circle A6 centre (-172, 103.08) radius 1.077
  circle A7 centre (-184.5, 103.08) radius 1.077
  line L20 (-153, 100.52) -> (-153, 101.92)
  line L21 (-153, 101.92) -> (-151, 101.92)
  line L22 (-151, 101.92) -> (-151, 100.52)
  line L23 (-151, 100.52) -> (-153, 100.52)
  line L24 (-164.46, 100.52) -> (-164.46, 101.92)
  line L25 (-164.46, 101.92) -> (-162.46, 101.92)
  line L26 (-162.46, 101.92) -> (-162.46, 100.52)
  line L27 (-162.46, 100.52) -> (-164.46, 100.52)
  arc A8 (-173.077, 97.105) -> (-172.975, 97.003) centre (-172.975, 97.105) ccw
  line L28 (-173.077, 97.105) -> (-173.077, 99.055)
  arc A9 (-172.975, 99.157) -> (-173.077, 99.055) centre (-172.975, 99.055) ccw
  line L29 (-172.975, 99.157) -> (-171.025, 99.157)
  arc A10 (-170.923, 99.055) -> (-171.025, 99.157) centre (-171.025, 99.055) ccw
  line L30 (-170.923, 99.055) -> (-170.923, 97.105)
  arc A11 (-171.025, 97.003) -> (-170.923, 97.105) centre (-171.025, 97.105) ccw
  line L31 (-171.025, 97.003) -> (-172.975, 97.003)
  circle A12 centre (-184.5, 98.08) radius 1.077
  line L32 (-153, 96.82) -> (-153, 98.22)
  line L33 (-153, 98.22) -> (-151, 98.22)
  line L34 (-151, 98.22) -> (-151, 96.82)
  line L35 (-151, 96.82) -> (-153, 96.82)
  line L36 (-164.46, 96.82) -> (-164.46, 98.22)
  line L37 (-164.46, 98.22) -> (-162.46, 98.22)
  line L38 (-162.46, 98.22) -> (-162.46, 96.82)
  line L39 (-162.46, 96.82) -> (-164.46, 96.82)
  line L40 (-212.43, 77.21) -> (-212.43, 78.91)
  line L41 (-212.43, 78.91) -> (-210.73, 78.91)
  line L42 (-210.73, 78.91) -> (-210.73, 77.21)
  line L43 (-210.73, 77.21) -> (-212.43, 77.21)
  circle A13 centre (-211.58, 75.52) radius 0.85
  circle A14 centre (-211.58, 72.98) radius 0.85
  circle A15 centre (-211.58, 70.44) radius 0.85
  circle A16 centre (-211.58, 67.9) radius 0.85
  circle A17 centre (-211.58, 65.36) radius 0.85
  circle A18 centre (-211.58, 62.82) radius 0.85
  circle A19 centre (-211.58, 60.28) radius 0.85
  circle A20 centre (-211.58, 57.74) radius 0.85
  circle A21 centre (-211.58, 55.2) radius 0.85
  circle A22 centre (-211.58, 52.66) radius 0.85
  circle A23 centre (-211.58, 50.12) radius 0.85
  circle A24 centre (-211.58, 47.58) radius 0.85
  circle A25 centre (-196.89, 46.1501) radius 0.6604
  circle A26 centre (-199.43, 46.1501) radius 0.6604
  circle A27 centre (-201.97, 46.1501) radius 0.6604
  circle A28 centre (-211.58, 45.04) radius 0.85
  circle A29 centre (-129.53, 40.19) radius 2.2
  circle A30 centre (-210.09, 40.19) radius 2.2
  circle A31 centre (-129.53, 102.8006) radius 2.1994
  circle A32 centre (-129.53, 102.8006) radius 1.0822
  dimension "d31" = -1.1172
  constraint tangent A4 A31
extrude "Extrude10" cut sketch "Sketch10" against normal blind 4.5 contours A32
sketch "Sketch11" plane through (0, 0, 1.56) normal (0, 0, 1) x (-1, 0, 0)
  arc A0 (-129.3118, 35.1924) -> (-124.5324, 39.9718) centre (-129.53, 40.19) ccw
  line L0 (-124.5324, 39.9718) -> (-124.53, 40.19)
  line L1 (-124.53, 40.19) -> (-124.53, 102.8)
  line L2 (-124.53, 102.8) -> (-124.5323, 103.0182)
  arc A1 (-124.5323, 103.0182) -> (-129.3118, 107.7977) centre (-129.53, 102.8) ccw
  line L3 (-129.3118, 107.7977) -> (-129.53, 107.8)
  line L4 (-129.53, 107.8) -> (-210.09, 107.8)
  line L5 (-210.09, 107.8) -> (-210.3082, 107.7977)
  arc A2 (-210.3082, 107.7977) -> (-215.0877, 103.0182) centre (-210.09, 102.8) ccw
  line L6 (-215.0877, 103.0182) -> (-215.09, 102.8)
  line L7 (-215.09, 102.8) -> (-215.09, 40.19)
  line L8 (-215.09, 40.19) -> (-215.0876, 39.9718)
  arc A3 (-215.0876, 39.9718) -> (-210.3082, 35.1924) centre (-210.09, 40.19) ccw
  line L9 (-210.3082, 35.1924) -> (-210.09, 35.19)
  line L10 (-210.09, 35.19) -> (-129.53, 35.19)
  line L11 (-129.53, 35.19) -> (-129.3118, 35.1924)
  circle A4 centre (-129.53, 102.8) radius 2.2
  circle A5 centre (-210.09, 102.8) radius 2.2
  line L12 (-153, 103.32) -> (-153, 104.72)
  line L13 (-153, 104.72) -> (-151, 104.72)
  line L14 (-151, 104.72) -> (-151, 103.32)
  line L15 (-151, 103.32) -> (-153, 103.32)
  line L16 (-164.46, 103.32) -> (-164.46, 104.72)
  line L17 (-164.46, 104.72) -> (-162.46, 104.72)
  line L18 (-162.46, 104.72) -> (-162.46, 103.32)
  line L19 (-162.46, 103.32) -> (-164.46, 103.32)
  circle A6 centre (-172, 103.08) radius 1.077
  circle A7 centre (-184.5, 103.08) radius 1.077
  line L20 (-153, 100.52) -> (-153, 101.92)
  line L21 (-153, 101.92) -> (-151, 101.92)
  line L22 (-151, 101.92) -> (-151, 100.52)
  line L23 (-151, 100.52) -> (-153, 100.52)
  line L24 (-164.46, 100.52) -> (-164.46, 101.92)
  line L25 (-164.46, 101.92) -> (-162.46, 101.92)
  line L26 (-162.46, 101.92) -> (-162.46, 100.52)
  line L27 (-162.46, 100.52) -> (-164.46, 100.52)
  arc A8 (-173.077, 97.105) -> (-172.975, 97.003) centre (-172.975, 97.105) ccw
  line L28 (-173.077, 97.105) -> (-173.077, 99.055)
  arc A9 (-172.975, 99.157) -> (-173.077, 99.055) centre (-172.975, 99.055) ccw
  line L29 (-172.975, 99.157) -> (-171.025, 99.157)
  arc A10 (-170.923, 99.055) -> (-171.025, 99.157) centre (-171.025, 99.055) ccw
  line L30 (-170.923, 99.055) -> (-170.923, 97.105)
  arc A11 (-171.025, 97.003) -> (-170.923, 97.105) centre (-171.025, 97.105) ccw
  line L31 (-171.025, 97.003) -> (-172.975, 97.003)
  circle A12 centre (-184.5, 98.08) radius 1.077
  line L32 (-153, 96.82) -> (-153, 98.22)
  line L33 (-153, 98.22) -> (-151, 98.22)
  line L34 (-151, 98.22) -> (-151, 96.82)
  line L35 (-151, 96.82) -> (-153, 96.82)
  line L36 (-164.46, 96.82) -> (-164.46, 98.22)
  line L37 (-164.46, 98.22) -> (-162.46, 98.22)
  line L38 (-162.46, 98.22) -> (-162.46, 96.82)
  line L39 (-162.46, 96.82) -> (-164.46, 96.82)
  line L40 (-212.43, 77.21) -> (-212.43, 78.91)
  line L41 (-212.43, 78.91) -> (-210.73, 78.91)
  line L42 (-210.73, 78.91) -> (-210.73, 77.21)
  line L43 (-210.73, 77.21) -> (-212.43, 77.21)
  circle A13 centre (-211.58, 75.52) radius 0.85
  circle A14 centre (-211.58, 72.98) radius 0.85
  circle A15 centre (-211.58, 70.44) radius 0.85
  circle A16 centre (-211.58, 67.9) radius 0.85
  circle A17 centre (-211.58, 65.36) radius 0.85
  circle A18 centre (-211.58, 62.82) radius 0.85
  circle A19 centre (-211.58, 60.28) radius 0.85
  circle A20 centre (-211.58, 57.74) radius 0.85
  circle A21 centre (-211.58, 55.2) radius 0.85
  circle A22 centre (-211.58, 52.66) radius 0.85
  circle A23 centre (-211.58, 50.12) radius 0.85
  circle A24 centre (-211.58, 47.58) radius 0.85
  circle A25 centre (-196.89, 46.1501) radius 0.6604
  circle A26 centre (-199.43, 46.1501) radius 0.6604
  circle A27 centre (-201.97, 46.1501) radius 0.6604
  circle A28 centre (-211.58, 45.04) radius 0.85
  circle A29 centre (-129.53, 40.19) radius 2.2
  circle A30 centre (-210.09, 40.19) radius 2.2
  circle A31 centre (-210.09, 40.1906) radius 2.1994
  circle A32 centre (-210.09, 40.1906) radius 1.0875
  dimension "d36" = -1.1119
  constraint tangent A30 A31
extrude "Extrude11" cut sketch "Sketch11" against normal blind 4.5 contours A32